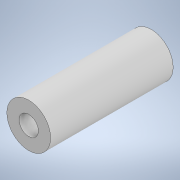
# Autodesk Inventor part: wały_sr
Saved by Autodesk Inventor 2022 (Build 260153000, 153)
## iProperties
Created: 2023-04-25
Part Number: wały_sr
Material: Ogólny
Document SubType Name: Modeling
Designer: nosal
Density: 1 g/cm^3
Appearance: Domyślna
Author: nosal
## iProperties of the stored document wały_sr_Drukowanie 3D.ipt
Created: 2023-05-07
Part Number: wały_sr_Drukowanie 3D
Material: Ogólny
Document SubType Name: Modeling
Designer: nosal
Density: 1 g/cm^3
Appearance: Domyślna
Author: nosal
Autodesk Inventor part; units mm, degrees
ref_plane "YZ Plane" through (0, 0, 0) normal (1, 0, 0) x (0, 1, 0)
ref_plane "XZ Plane" through (0, 0, 0) normal (0, 1, 0) x (-1, 0, 0)
ref_plane "XY Plane" through (0, 0, 0) normal (0, 0, 1) x (1, 0, 0)
sketch "Szkic1" plane through (0, 0, 0) normal (0, 0, 1) x (1, 0, 0)
  circle A0 centre (0, 0) radius 25
  circle A1 centre (0, 0) radius 11
  dimension "d1" = 50
  dimension "d2" = 22
  constraints: 2 centre point, 2 coincident
  measures "d1" diameter of A0
  measures "d2" diameter of A1
extrude "Wyciągnięcie proste1" add sketch "Szkic1" along normal blind 140
